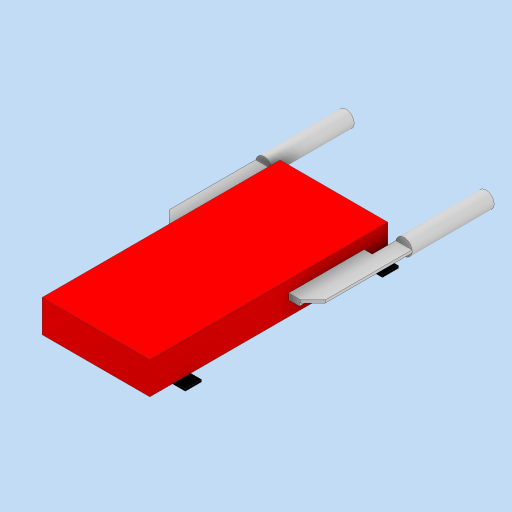
# Autodesk Inventor part: CO-1-1_BMS
Saved by Autodesk Inventor 2023 (Build 270158000, 158)
## iProperties
Created: 2023-01-21
Part Number: CO-1-1_BMS
Material: Generic
Document SubType Name: Modeling
Designer: asach
Density: 1 g/cm^3
Appearance: Default
Author: asach
Autodesk Inventor part; units mm, degrees
ref_plane "YZ Plane" through (0, 0, 0) normal (1, 0, 0) x (0, 1, 0)
ref_plane "XZ Plane" through (0, 0, 0) normal (0, 1, 0) x (-1, 0, 0)
ref_plane "XY Plane" through (0, 0, 0) normal (0, 0, 1) x (1, 0, 0)
sketch "Sketch1" plane through (0, 0, 0) normal (0, 1, 0) x (-1, 0, 0)
  line L0 (0, 0) -> (100, 0)
  line L1 (100, 0) -> (100, -221)
  line L2 (100, -221) -> (0, -221)
  line L3 (0, -221) -> (0, 0)
  dimension "d0" = 100
  dimension "d1" = 221
  constraints: 8 end point, 2 parallel, 1 horizontal, 1 perpendicular
  measures "d0" distance of L1.end L2.end
  measures "d1" distance of L0.end L1.end
extrude "Extrusion1" add sketch "Sketch1" along normal blind 30
sketch "Sketch2" plane through (0, 0, 0) normal (0, -1, 0) x (1, 0, 0)
  line L0 (-110, -23) -> (10, -23)
  line L1 (10, -23) -> (10, -38)
  line L2 (10, -38) -> (-110, -38)
  line L3 (-110, -38) -> (-110, -23)
  line L4 (-110, -206) -> (10, -206)
  line L5 (10, -206) -> (10, -221)
  line L6 (10, -221) -> (-110, -221)
  line L7 (-110, -221) -> (-110, -206)
  line L8 (-100, 0) -> (0, 0) projected
  line L9 (-50, -23) -> (-50, -38) construction
  line L10 (-100, 0) -> (0, 0) projected
  line L11 (-50, 0) -> (-50, -221) construction
  line L12 (0, -221) -> (-100, -221) projected
  line L13 (0, -221) -> (-100, -221) projected
  dimension "d4" = 23
  dimension "d5" = 15
  dimension "d6" = 120
  constraints: 20 end point, 4 midpoint, 4 parallel, 3 collinear, 2 equal length, 2 horizontal, 2 perpendicular
  measures "d4" distance between parallel lines of L8 L0
  measures "d5" distance of L0.end L1.end
  measures "d6" distance of L0.start L0.end
extrude "Extrusion2" add sketch "Sketch2" along normal blind 2
ref_plane "Work Plane1" through (0, 15, 0) normal (0, 1, 0) x (1, 0, 0)
sketch "Sketch3" plane through (0, 0, 0) normal (0, 1, 0) x (-1, 0, 0)
  line L0 (0, 0) -> (0, -221) projected
  line L1 (0, -38) -> (0, -206) projected
  line L2 (0, -199) -> (-10, -199)
  line L3 (-10, -199) -> (-10, -129)
  line L4 (-10, -129) -> (0, -129)
  line L5 (0, -129) -> (0, -199)
  line L6 (0, -221) -> (100, -221) projected
  dimension "d9" = 22
  dimension "d10" = 10
  dimension "d11" = 70
  constraints: 8 end point, 2 parallel, 1 horizontal, 1 perpendicular, 1 point on line
  measures "d9" distance between parallel lines of L6 L2
  measures "d10" distance of L3.end L4.end
  measures "d11" distance of L2.end L3.end
extrude "Extrusion3" add sketch "Sketch3" along normal mid plane 3 from surface at 15
ref_plane "Work Plane2" through (-50, 0, 0) normal (1, 0, 0) x (0, 0, -1)
mirror "Mirror1" about plane through (-50, 0, 0) normal (1, 0, 0) of "Extrusion3"
sketch "Sketch4" plane through (0, 16.5, -129) normal (0, 1, 0) x (1, 0, 0)
  line L0 (10, 0) -> (0, 0) projected
  line L1 (10, 70) -> (10, 0) projected
  line L2 (0, 70) -> (10, 70) projected
  line L3 (0, 0) -> (0, 70) projected
  line L4 (0, 70) -> (10, 70)
  line L5 (0, 70) -> (0, 0)
  line L6 (0, -129) -> (0, 92) projected
  line L7 (0, 0) -> (11, 0)
  line L8 (22.5, 11.5) -> (22.5, 70)
  line L9 (0, 70) -> (7.5, 70)
  line L10 (11, 0) -> (22.5, 11.5)
  line L11 (7.5, 70) -> (10, 70)
  line L12 (22.5, 70) -> (22.5, 92)
  line L13 (22.5, 92) -> (7.5, 92)
  line L14 (7.5, 92) -> (7.5, 70)
  dimension "d17" = 22.5
  dimension "d19" = 45
  dimension "d20" = 11
  dimension "d23" = 7.5
  dimension "d24" = 22
  constraints: 20 end point, 2 horizontal, 2 parallel, 2 perpendicular, 1 collinear, 1 point on line
  measures "d17" distance of L2.start L8.end
  measures "d19" angle of L7 L10
  measures "d20" distance from line of L7.end L3
  measures "d23" distance between parallel lines of L14 L6
  measures "d24" distance of L12.start L12.end
extrude "Extrusion4" add sketch "Sketch4" along normal blind 2.5
mirror "Mirror2" about plane through (-50, 0, 0) normal (1, 0, 0) of "Extrusion4"
ref_plane "Work Plane4" through (15, 16.5, -140.5) normal (1, 0, 0) x (0, 0, -1)
ref_plane "Work Plane3" through (0, 17.75, -129) normal (0, 1, 0) x (1, 0, 0)
sketch "Sketch5" plane through (22.5, 16.5, -221) normal (0, 0, -1) x (-1, 0, 0)
  circle A0 centre (7.5, 1.25) radius 7.5011
  line L0 (7.5, -24.9) -> (7.5, 19.9) projected
  line L1 (-29.0013, 1.25) -> (174.0002, 1.25) projected
  point P0 (22.5, -16.5)
  dimension "d25" = 0
  dimension "d26" = 0
  constraints: 1 centre point
  measures "d25" distance from line of L0 A0.centre
  measures "d26" distance from line of L1 A0.centre
extrude "Extrusion5" add sketch "Sketch5" along normal blind 76.2
mirror "Mirror3" about plane through (-50, 0, 0) normal (1, 0, 0) of "Extrusion5"
body "Solid1"
